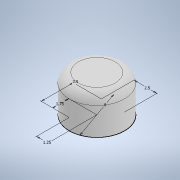
# Autodesk Inventor part: Power_Button
Saved by Autodesk Inventor 2021 (Build 250183000, 183)
## iProperties
Created: 2020-08-18
Part Number: Power_Button
Material: Generic
Document SubType Name: Modeling
Designer: ridvansong
Density: 1 g/cm^3
Appearance: Default
Author: ridvansong
Autodesk Inventor part; units mm, degrees
ref_plane "YZ Plane" through (0, 0, 0) normal (1, 0, 0) x (0, 1, 0)
ref_plane "XZ Plane" through (0, 0, 0) normal (0, 1, 0) x (-1, 0, 0)
ref_plane "XY Plane" through (0, 0, 0) normal (0, 0, 1) x (1, 0, 0)
sketch "Sketch1" plane through (0, 0, 0) normal (0, 1, 0) x (-1, 0, 0)
  circle A0 centre (0, 0) radius 3
  line L0 (1.25, 1.75) -> (-1.25, 1.75)
  line L1 (-1.25, 1.75) -> (-1.25, -1.75)
  line L2 (-1.25, -1.75) -> (1.25, -1.75)
  line L3 (1.25, -1.75) -> (1.25, 1.75)
  dimension "d0" = 6
  dimension "d1" = 2.5
  dimension "d2" = 3.5
  dimension "d3" = 1.25
  dimension "d4" = 1.75
  constraints: 8 end point, 2 parallel, 1 centre point, 1 coincident, 1 horizontal, 1 perpendicular
  measures "d0" diameter of A0
  measures "d1" distance between parallel lines of L1 L3
  measures "d2" distance between parallel lines of L2 L0
  measures "d3" distance from line of point (0, 0) L3
  measures "d4" distance from line of point (0, 0) L0
extrude "Extrusion1" add sketch "Sketch1" along normal blind 4 contours A0 | L3 L2 L1 L0
extrude "Extrusion2" cut sketch "Sketch1" along normal blind 3 contours L3 L2 L1 L0
fillet "Fillet1" radius 1 1 edges at (3, 4, 0)
body "Solid1"
